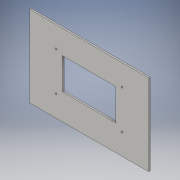
# Autodesk Inventor part: Lock
Saved by Autodesk Inventor 2016 SP2 (Build 200236200, 236)
## iProperties
Created: 2017-08-28
Part Number: Lock
Material: Generic
Document SubType Name: Modeling
Designer: Albin Hjalmas
Density: 1 g/cm^3
Appearance: Default
Author: Albin Hjalmas
Autodesk Inventor part; units mm, degrees
ref_plane "YZ Plane" through (0, 0, 0) normal (1, 0, 0) x (0, 1, 0)
ref_plane "XZ Plane" through (0, 0, 0) normal (0, 1, 0) x (-1, 0, 0)
ref_plane "XY Plane" through (0, 0, 0) normal (0, 0, 1) x (1, 0, 0)
sketch "Sketch1" plane through (0, 0, 0) normal (0, 0, 1) x (1, 0, 0)
  line L0 (0, 0) -> (220, 0)
  line L1 (220, 0) -> (220, 150)
  line L2 (220, 150) -> (0, 150)
  line L3 (0, 150) -> (0, 0)
  dimension "d0" = 220
  dimension "d1" = 150
  constraints: 8 end point, 2 parallel, 1 horizontal, 1 perpendicular
  measures "d0" distance of L2.end L1.end
  measures "d1" distance of L1.end L0.end
extrude "Extrusion1" add sketch "Sketch1" along normal blind 3
sketch "Sketch2" plane through (0, 0, 3) normal (0, 0, 1) x (1, 0, 0)
  line L0 (0, 150) -> (0, 0) projected
  line L1 (0, 75) -> (220, 75)
  line L2 (220, 0) -> (220, 150) projected
  line L3 (220, 150) -> (0, 150) projected
  line L4 (110, 150) -> (110, 0)
  circle A0 centre (49, 111) radius 1.6
  circle A1 centre (171, 111) radius 1.6
  circle A2 centre (171, 39) radius 1.6
  circle A3 centre (49, 39) radius 1.6
  line L5 (60.5, 48) -> (159.5, 48)
  line L6 (159.5, 48) -> (159.5, 106)
  line L7 (159.5, 106) -> (60.5, 106)
  line L8 (60.5, 106) -> (60.5, 48)
  dimension "d7" = 3.2
  dimension "d8" = 3.2
  dimension "d9" = 3.2
  dimension "d10" = 3.2
  dimension "d11" = 99
  dimension "d12" = 58
  dimension "d13" = 11.5
  dimension "d14" = 5
  dimension "d15" = 9
  constraints: 12 end point, 4 centre point, 3 midpoint, 2 parallel, 1 horizontal, 1 perpendicular, 1 vertical
  measures "d7" diameter of A0
  measures "d8" diameter of A1
  measures "d9" diameter of A2
  measures "d10" diameter of A3
  measures "d11" distance of L7.end L6.end
  measures "d12" distance of L6.end L5.end
  measures "d13" distance from line of A1.centre L6
  measures "d14" distance from line of A1.centre L7
  measures "d15" distance from line of A2.centre L5
sketch "Sketch3" plane through (0, 0, 3) normal (0, 0, 1) x (1, 0, 0)
  circle A0 centre (49, 111) radius 1.6
  circle A1 centre (171, 111) radius 1.6
  circle A2 centre (171, 39) radius 1.6
  circle A3 centre (49, 39) radius 1.6
  line L0 (60.5, 48) -> (159.5, 48)
  line L1 (159.5, 48) -> (159.5, 106)
  line L2 (159.5, 106) -> (60.5, 106)
  line L3 (60.5, 106) -> (60.5, 48)
  point P0 (0, 0)
  dimension "d16" = 3.2
  dimension "d17" = 3.2
  dimension "d18" = 3.2
  dimension "d19" = 3.2
  dimension "d20" = 99
  dimension "d21" = 58
  dimension "d22" = 11.5
  dimension "d23" = 5
  dimension "d24" = 9
  constraints: 8 end point, 4 centre point, 2 parallel, 1 horizontal, 1 perpendicular
  measures "d16" diameter of A0
  measures "d17" diameter of A1
  measures "d18" diameter of A2
  measures "d19" diameter of A3
  measures "d20" distance of L2.end L2.start
  measures "d21" distance of L2.start L0.end
  measures "d22" distance from line of A1.centre L1
  measures "d23" distance from line of A1.centre L2
  measures "d24" distance from line of A2.centre L0
extrude "Extrusion2" cut sketch "Sketch3" against normal blind 3
body "Solid1"
